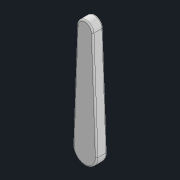
# Autodesk Inventor part: link3
Saved by Autodesk Inventor 2021 (Build 250183000, 183)
## iProperties
Created: 2021-07-10
Part Number: link3
Material: 一般
Document SubType Name: Modeling
Designer: yuta0
Density: 1 g/cm^3
Appearance: 既定
Author: yuta0
Autodesk Inventor part; units mm, degrees
ref_plane "YZ Plane" through (0, 0, 0) normal (1, 0, 0) x (0, 1, 0)
ref_plane "XZ Plane" through (0, 0, 0) normal (0, 1, 0) x (-1, 0, 0)
ref_plane "XY Plane" through (0, 0, 0) normal (0, 0, 1) x (1, 0, 0)
sketch "スケッチ1" plane through (0, 0, 0) normal (0, 0, 1) x (1, 0, 0)
  circle A0 centre (0, 0) radius 45
  circle A1 centre (0, 400) radius 30
  line L0 (-29.9789, 401.125) -> (-44.9683, 1.6875)
  line L1 (44.9683, 1.6875) -> (29.9789, 401.125)
  dimension "d0" = 90
  dimension "d1" = 60
  dimension "d2" = 400
  constraints: 4 end point, 4 point on circle, 4 tangent, 2 centre point, 1 coincident, 1 vertical alignment
  measures "d0" diameter of A0
  measures "d1" diameter of A1
  measures "d2" distance of A0.centre A1.centre
extrude "押し出し1" add sketch "スケッチ1" along normal mid plane 40
fillet "フィレット1" radius 5 8 edges at (0, 430, -20) (37.4736, 201.4062, -20) (0, -45, -20) (-37.4736, 201.4062, -20) (0, -45, 20) (37.4736, 201.4062, 20) (0, 430, 20) (-37.4736, 201.4062, 20)
